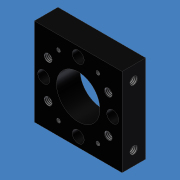
# Autodesk Inventor part: BB1-FrontPlate
Saved by Autodesk Inventor 2015 (Build 190159000, 159)
## iProperties
Company: FirstCadLibrary
Shininess: 64.0
Length Units: 11269
Angle Units: 11279
Time Units: 11290
Mass Units: 11283
Length Display Precision: 3
Angle Display Precision: 2
Compacted: True
Part Number: BB1-FrontPlate
Document SubType Name: Modeling
Created: 2007-01-08
Material: Steel, Mild
Designer: Ed Sparks
Catalog Web Link: www.banebots.com
Vendor: BaneBots
Density: 1 g/cm^3
Appearance: Anodized - Black
Density: 0.0
Volumn: 0.0
Area: 0.0
PropertySet Name: Model Information
Control State: 0
Master: False
Checked Out: False
Author: Ed Sparks
Autodesk Inventor part; units mm, degrees
ref_plane "YZ Plane" through (0, 0, 0) normal (1, 0, 0) x (0, 1, 0)
ref_plane "XZ Plane" through (0, 0, 0) normal (0, 1, 0) x (-1, 0, 0)
ref_plane "XY Plane" through (0, 0, 0) normal (0, 0, 1) x (1, 0, 0)
sketch "Sketch1" plane through (0, 0, 0) normal (0, 0, 1) x (1, 0, 0)
  line L0 (-22.225, 22.225) -> (22.225, 22.225)
  line L1 (22.225, 22.225) -> (22.225, -22.225)
  line L2 (22.225, -22.225) -> (-22.225, -22.225)
  line L3 (-22.225, -22.225) -> (-22.225, 22.225)
  line L4 (0, 0) -> (0, 22.225) construction
  line L5 (0, 0) -> (0, -22.225) construction
  line L6 (0, 0) -> (22.225, 0) construction
  line L7 (0, 0) -> (-22.225, 0) construction
  dimension "d0" = 44.45
  dimension "d1" = 44.45
  constraints: 16 end point, 4 midpoint, 3 perpendicular, 2 collinear, 2 parallel, 1 horizontal, 1 other
  measures "d0" distance of L0.start L0.end
  measures "d1" distance of L0.end L1.end
extrude "Extrusion1" add sketch "Sketch1" along normal mid plane 11.938
sketch "Sketch2" plane through (0, 0, -5.969) normal (0, 0, -1) x (-1, 0, 0)
  point P0 (0, 0)
  constraints: 1 other
hole "Hole1" at (0, 0, -5.969) direction (0, 0, 1) diameter 22 end through all
sketch "Sketch3" plane through (0, 0, -5.969) normal (0, 0, -1) x (-1, 0, 0)
  circle A0 centre (0, 0) radius 11 projected
  point P0 (0, 17.5)
  dimension "d11" = 17.5
  constraints: 1 vertical alignment
  measures "d11" distance of point (0, 17.5) A0.centre
hole "Hole2" at (0, 17.5, -5.969) direction (0, 0, 1) diameter 3.4 end through all counterbore diameter 6 counterbore depth 5.5
pattern_circular "Circular Pattern1" count 4 over 360 about axis through (0, 0, 58.0163) along (0, 0, -1) of "Hole2"
sketch "Sketch4" plane through (0, 0, -5.969) normal (0, 0, -1) x (-1, 0, 0)
  circle A0 centre (0, 0) radius 11 projected
  circle A1 centre (0, 17.5) radius 3 projected
  point P0 (-9.525, 15.24)
  dimension "d22" = 15.24
  dimension "d49" = 9.525
  measures "d22" vertical distance of point (-9.525, 15.24) A0.centre
  measures "d49" horizontal distance of A1.centre point (-9.525, 15.24)
hole "Hole3" at (9.525, 15.24, -5.969) direction (0, 0, 1) diameter 3.962 end through all thread size "10-32 UNF" class "2B" standard "ANSI Unified Screw Threads"
mirror "Mirror1" about plane through (0, 0, 0) normal (1, 0, 0) of "Hole3"
mirror "Mirror2" about plane through (0, 0, 0) normal (0, 1, 0) of "Hole3", "Mirror1"
sketch "Sketch5" plane through (0, 0, -5.969) normal (0, 0, -1) x (-1, 0, 0)
  circle A0 centre (0, 0) radius 11 projected
  point P0 (-15.5, 10)
  dimension "d31" = 10
  dimension "d32" = 15.5
  measures "d31" vertical distance of point (-15.5, 10) A0.centre
  measures "d32" horizontal distance of point (-15.5, 10) A0.centre
hole "Hole4" at (15.5, 10, -5.969) direction (0, 0, 1) diameter 2.013 end through all thread size "M2.5x0.45" class "6H" standard "ANSI Metric M Profile"
mirror "Mirror3" about plane through (0, 0, 0) normal (0, 1, 0) of "Hole4"
mirror "Mirror4" about plane through (0, 0, 0) normal (1, 0, 0) of "Hole4", "Mirror3", "Hole1"
sketch "Sketch6" plane through (-22.225, 22.225, 5.969) normal (0, 1, 0) x (1, 0, 0)
  line L0 (0, 0) -> (44.45, 0) projected
  line L1 (44.45, 11.938) -> (0, 11.938) projected
  line L2 (22.225, 0) -> (22.225, 11.938) construction
  line L3 (44.45, 0) -> (44.45, 11.938) projected
  line L4 (0, 11.938) -> (0, 0) projected
  line L5 (0, 5.969) -> (44.45, 5.969) construction
  point P0 (37.465, 5.969)
  dimension "d41" = 15.24
  constraints: 4 end point, 4 midpoint, 1 point on line
  measures "d41" horizontal distance of point (37.465, 5.969) L2.end
hole "Hole5" at (15.24, 22.225, 0) direction (0, -1, 0) diameter 3.962 depth 6 tip angle 118 thread size "10-32 UNF" class "2B" standard "ANSI Unified Screw Threads"
mirror "Mirror5" about plane through (0, 0, 0) normal (1, 0, 0) of "Hole5"
mirror "Mirror6" about plane through (0, 0, 0) normal (0, 1, 0) of "Hole5", "Mirror5"
body "Solid1"
